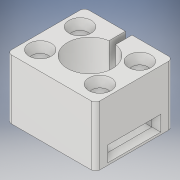
# Autodesk Inventor part: Electromagnet Blocl
Saved by Autodesk Inventor 2019 (Build 230136000, 136)
## iProperties
Created: 2018-12-14
Part Number: Electromagnet Blocl
Material: ABS Plastic
Document SubType Name: Modeling
Designer: Ax
Density: 1.06 g/cm^3
Appearance: Smooth - White
Author: Ax
Autodesk Inventor part; units mm, degrees
ref_plane "YZ Plane" through (0, 0, 0) normal (1, 0, 0) x (0, 1, 0)
ref_plane "XY Plane" through (0, 0, 0) normal (0, 0, 1) x (1, 0, 0)
sketch "Sketch1" plane through (0, 0, 0) normal (0, 1, 0) x (-1, 0, 0)
  line L0 (-20, 17.5) -> (20, 17.5)
  line L1 (20, 17.5) -> (20, -17.5)
  line L2 (20, -17.5) -> (-20, -17.5)
  line L3 (-20, -17.5) -> (-20, 17.5)
  line L4 (-20, 17.5) -> (20, -17.5) construction
  line L5 (20, 17.5) -> (-20, -17.5) construction
  point P0 (0, 0)
  dimension "d0" = 35
  dimension "d1" = 40
  constraints: 12 end point, 2 midpoint, 2 parallel, 1 horizontal, 1 perpendicular
  measures "d0" distance of L2.end L0.start
  measures "d1" distance of L1.end L2.end
extrude "Extrusion1" add sketch "Sketch1" along normal blind 21
sketch "Sketch2" plane through (0, 21, 0) normal (0, 1, 0) x (1, 0, 0)
  circle A0 centre (0, 0) radius 10.2
  line L0 (-1.5, 10.0891) -> (-1.5, 17.5)
  line L1 (-1.5, 17.5) -> (1.5, 17.5)
  line L2 (20, 17.5) -> (-20, 17.5) projected
  line L3 (1.5, 17.5) -> (1.5, 10.0891)
  line L4 (0, 0) -> (0, 17.5) construction
  dimension "d4" = 20.4
  dimension "d7" = 3
  constraints: 8 end point, 2 point on circle, 1 centre point, 1 coincident, 1 midpoint, 1 perpendicular, 1 point on line, 1 symmetric about line, 1 vertical
  measures "d4" diameter of A0
  measures "d7" distance between parallel lines of L3 L0
extrude "Extrusion2" cut sketch "Sketch2" against normal blind 15
sketch "Sketch3" plane through (0, 6, 0) normal (0, 1, 0) x (1, 0, 0)
  circle A0 centre (0, 0) radius 2.25
  dimension "d8" = 4.5
  constraints: 1 centre point, 1 coincident
  measures "d8" diameter of A0
extrude "Extrusion3" cut sketch "Sketch3" against normal through all
sketch "Sketch5" plane through (0, 0, 0) normal (0, -1, 0) x (1, 0, 0)
  circle A0 centre (0, 0) radius 7.25
  dimension "d11" = 14.5
  constraints: 1 centre point, 1 coincident
  measures "d11" diameter of A0
extrude "Extrusion4" cut sketch "Sketch5" against normal blind 3
sketch "Sketch6" plane through (0, 21, 0) normal (0, 1, 0) x (1, 0, 0)
  line L0 (-13.5, -9) -> (13.5, -9) construction
  line L1 (13.5, -9) -> (13.5, 9) construction
  line L2 (13.5, 9) -> (-13.5, 9) construction
  line L3 (-13.5, 9) -> (-13.5, -9) construction
  line L4 (-13.5, -9) -> (13.5, 9) construction
  line L5 (13.5, -9) -> (-13.5, 9) construction
  circle A0 centre (-13.5, 9) radius 5.05
  circle A1 centre (13.5, 9) radius 5.05
  circle A2 centre (13.5, -9) radius 5.05
  circle A3 centre (-13.5, -9) radius 5.05
  point P0 (0, 0)
  dimension "d14" = 18
  dimension "d15" = 27
  dimension "d16" = 10.1
  constraints: 12 end point, 4 centre point, 4 coincident, 3 equal radius, 2 midpoint, 2 parallel, 1 horizontal, 1 perpendicular
  measures "d14" distance of L1.end L0.end
  measures "d15" distance of L1.end L2.end
  measures "d16" diameter of A1
ref_plane "Work Plane1" through (0, 17, 0) normal (0, 1, 0) x (-1, 0, 0)
sketch "Sketch7" plane through (0, 17, 0) normal (0, 1, 0) x (-1, 0, 0)
  circle A0 centre (13.5, -9) radius 3.65
  circle A1 centre (-13.5, -9) radius 3.65
  circle A2 centre (-13.5, 9) radius 3.65
  circle A3 centre (13.5, 9) radius 3.65
  line L0 (13.5, 9) -> (-13.5, 9) construction
  line L1 (-13.5, 9) -> (-13.5, -9) construction
  line L2 (-13.5, -9) -> (13.5, -9) construction
  line L3 (13.5, -9) -> (13.5, 9) construction
  line L4 (13.5, 9) -> (-13.5, -9) construction
  line L5 (-13.5, 9) -> (13.5, -9) construction
  point P0 (0, 0)
  dimension "d20" = 7.3
  dimension "d21" = 27
  dimension "d22" = 18
  constraints: 12 end point, 4 centre point, 4 coincident, 3 equal radius, 2 midpoint, 2 parallel, 1 horizontal, 1 perpendicular
  measures "d20" diameter of A1
  measures "d21" distance of L0.start L0.end
  measures "d22" distance of L0.end L1.end
loft "Loft2" cut profiles "Sketch6", "Sketch7" contours A0 / A0
loft "Loft3" cut profiles "Sketch6", "Sketch7" contours A3 / A3
loft "Loft4" cut profiles "Sketch6", "Sketch7" contours A1 / A1
loft "Loft5" cut profiles "Sketch6", "Sketch7" contours A2 / A2
sketch "Sketch8" plane through (0, 0, 0) normal (0, -1, 0) x (1, 0, 0)
  line L0 (-20, -17.5) -> (20, -17.5)
  line L1 (20, -17.5) -> (20, -10)
  line L2 (-20, -10) -> (-20, -17.5)
  line L3 (-20, 17.5) -> (20, 17.5)
  line L4 (20, 17.5) -> (20, 10)
  line L5 (-20, 10) -> (-20, 17.5)
  line L6 (20, 10) -> (-20, 10)
  line L7 (20, -10) -> (-20, -10)
  point P0 (0, 0)
  dimension "d50" = 20
  constraints: 16 end point, 4 parallel, 2 coincident, 2 horizontal, 2 perpendicular, 1 collinear
  measures "d50" distance between parallel lines of L6 L7
extrude "Extrusion6" add sketch "Sketch8" along normal blind 3
sketch "Sketch9" plane through (0, -3, 0) normal (0, -1, 0) x (1, 0, 0)
  line L0 (-20, 17.5) -> (20, 17.5) projected
  line L1 (-20, -17.5) -> (-20, 17.5) projected
  line L2 (20, 17.5) -> (-20, 17.5)
  line L3 (-20, 17.5) -> (-20, -17.5)
  line L4 (-20, -17.5) -> (20, -17.5)
  line L5 (20, -17.5) -> (20, 17.5)
  circle A0 centre (0, 0) radius 7.25
  arc A1 (7.25, 0) -> (7.25, 0) centre (0, 0) ccw projected
  constraints: 8 end point, 2 parallel, 1 centre point, 1 coincident, 1 concentric, 1 horizontal, 1 perpendicular
extrude "Extrusion7" add sketch "Sketch9" along normal blind 3
fillet "Fillet1" radius 2 4 edges at (-20, 7.5, -17.5) (-20, 7.5, 17.5) (20, 7.5, -17.5) (20, 7.5, 17.5)
chamfer "Chamfer1" distance 2 angle 45 8 edges at (-20, -3, 0) (-20, -1.5, -10) (-20, 0, 0) (-20, -1.5, 10) (20, 0, 0) (20, -1.5, 10) (20, -3, 0) (20, -1.5, -10)
sketch "Sketch10" plane through (0, -6, 0) normal (0, -1, 0) x (1, 0, 0)
  line L0 (10, 12.5) -> (-10, 12.5) construction
  line L1 (-10, 12.5) -> (-10, -12.5) construction
  line L2 (-10, -12.5) -> (10, -12.5) construction
  line L3 (10, -12.5) -> (10, 12.5) construction
  line L4 (10, 12.5) -> (-10, -12.5) construction
  line L5 (-10, 12.5) -> (10, -12.5) construction
  circle A0 centre (10, -12.5) radius 2
  circle A1 centre (10, 12.5) radius 2
  circle A2 centre (-10, 12.5) radius 2
  circle A3 centre (-10, -12.5) radius 2
  point P0 (0, 0)
  dimension "d55" = 20
  dimension "d56" = 25
  dimension "d57" = 4
  constraints: 12 end point, 4 centre point, 4 coincident, 3 equal radius, 2 midpoint, 2 parallel, 1 horizontal, 1 perpendicular
  measures "d55" distance of L1.end L2.end
  measures "d56" distance of L0.end L1.end
  measures "d57" diameter of A0
extrude "Extrusion8" cut sketch "Sketch10" against normal blind 10
body "Solid1"
